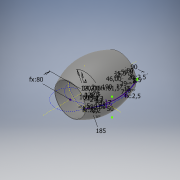
# Autodesk Inventor part: Form
Saved by Autodesk Inventor 2018.3 (Build 223284000, 284)
## iProperties
Created: 2018-07-22
Part Number: Form
Material: Generisch
Document SubType Name: Modeling
Designer: JochenAlt
Density: 1 g/cm^3
Appearance: Textur - grau
Author: JochenAlt
Autodesk Inventor part; units mm, degrees
ref_plane "YZ Plane" through (0, 0, 0) normal (1, 0, 0) x (0, 1, 0)
ref_plane "XY Plane" through (0, 0, 0) normal (0, 0, 1) x (1, 0, 0)
sketch "Skizze3" plane through (0, 0, 0) normal (0, 0, 1) x (1, 0, 0)
  line L0 (0, 284.3849) -> (0, -234.0642) construction
  line L1 (-127.25, 0) -> (203.5, 0) construction
  line L2 (92.5, 190) -> (90, 190)
  circle A0 centre (0, 0) radius 80 construction
  circle A1 centre (0, -80) radius 80 construction
  line L3 (83, -80) -> (85.5, -80)
  line L4 (83, -80) -> (131.774, 9.2102) construction
  line L5 (131.774, 94.6678) -> (90, 190) construction
  spline S0 degree 3 poles (83, -80) (131.774, 9.2102) (131.774, 94.6678) (90, 190) knots 1 1 1 1 2 2 2 2
  line L6 (92.5, 190) -> (133.774, 95.8088) construction
  line L7 (133.774, 8.2956) -> (85.5, -80) construction
  spline S1 degree 3 poles (92.5, 190) (133.774, 95.8088) (133.774, 8.2956) (85.5, -80) knots 1 1 1 1 2 2 2 2
  line L8 (153.75, 101.6438) -> (156.25, 101.6438) construction
  line L9 (153.75, 101.6438) -> (156.25, 101.6438) construction
  line L10 (133.774, 95.8088) -> (133.774, 8.2956) construction
  line L11 (131.774, 9.2102) -> (131.774, 94.6678) construction
  line L12 (57.5472, 55.5727) -> (101.7866, 98.2942) construction
  line L13 (57.5472, -24.4273) -> (101.7866, 18.2942) construction
  circle A2 centre (101.7866, 18.2942) radius 8.5 construction
  circle A3 centre (101.7866, 98.2942) radius 8.5 construction
  line L14 (83, -80) -> (80, -80) construction
  line L15 (110.1767, 16.9319) -> (117.0862, 15.81) construction
  line L16 (110.1836, 99.6135) -> (117.0987, 100.7) construction
  line L17 (109.0162, 129.7466) -> (110.9529, 130.2457) construction
  arc A4 (104.9108, 115.2128) -> (105.281, 136.4227) centre (94.4909, 126.0029) ccw construction
  line L18 (105.281, 136.4227) -> (51.2009, 192.4243) construction
  line L19 (104.9108, 115.2128) -> (67.4188, 79.0073) construction
  line L20 (92.5, 190) -> (88.2437, 199.7132) construction
  line L21 (88.2437, 199.7132) -> (82.5, 210) construction
  spline S2 degree 2 poles (92.5, 190) (88.2437, 199.7132) (82.5, 210) knots 1 1 1 2 2 2
  line L22 (90, 190) -> (85.7437, 199.7132) construction
  line L23 (85.7437, 199.7132) -> (80, 210) construction
  spline S3 degree 2 poles (90, 190) (85.7437, 199.7132) (80, 210) knots 1 1 1 2 2 2
  line L24 (82.5, 210) -> (80, 210)
  line L25 (90, 190) -> (90, 185)
  line L26 (90, 185) -> (88, 185)
  line L27 (88, 185) -> (88, 183)
  line L28 (88, 183) -> (92.9995, 183)
  line L29 (90, 190) -> (59.8, 190) construction
  line L30 (59.8, 190) -> (59.8, 185)
  line L31 (59.8, 185) -> (22, 172.5)
  arc A5 (49.9582, 183.7454) -> (59.8, 190) centre (42.4636, 206.409) ccw
  line L32 (49.9582, 183.7454) -> (22, 174.5)
  line L33 (22, 174.5) -> (22, 172.5)
  line L34 (59.8, 185) -> (88, 185) construction
  line L35 (22, 174.5) -> (9.0124, 174.5)
  line L36 (9.0124, 174.5) -> (9.0124, 172.5)
  line L37 (9.0124, 172.5) -> (22, 172.5)
  point P0 (90, 149.8145)
  point P1 (22, 173.5)
  dimension "d13" = 160
  dimension "d108" = 17
  dimension "d7" = 190
  dimension "d11" = 2.5
  dimension "d14" = 80
  dimension "d15" = 90
  dimension "d18" = 2.5
  dimension "d19" = 2.5
  dimension "d105" = 2
  dimension "d106" = 61.5
  dimension "d107" = 46
  dimension "d110" = 3
  dimension "d111" = 7
  dimension "d112" = 7
  dimension "d119" = 10
  dimension "d120" = 15
  dimension "d121" = 29
  dimension "d122" = 2
  dimension "d127" = 2.5
  dimension "d128" = 80
  dimension "d129" = 20
  dimension "d137" = 5
  dimension "d149" = 2
  dimension "d181" = 2
  dimension "d183" = 59.8
  dimension "d184" = 22
  dimension "d185" = 15.5
  constraints: 52 end point, 10 horizontal, 9 point on circle, 8 parallel, 5 point on line, 4 perpendicular, 3 centre point, 3 equal length, 3 tangent, 3 vertical, 2 coincident, 2 line through centre, 1 collinear, 1 midpoint, 31 other
  measures "d7" distance between parallel lines of L1 L2
  measures "d11" distance of L2.start L2.end
  measures "d14" distance of A1.centre point (0, 0)
  measures "d15" distance from line of L0 L2.end
  measures "d18" distance of L3.end L3.start
  measures "d19" distance of L8.start L8.end
  measures "d105" distance between parallel lines of L10 L11
  measures "d106" distance of L12.start L12.end
  measures "d107" angle of L0 L12
  measures "d110" distance of L3.start L14.end
  measures "d111" distance of L15.start L15.end
  measures "d112" distance of L16.start L16.end
  measures "d119" distance from line of L19.start L12
  measures "d120" radius of A4
  measures "d121" distance from line of L18 point (101.787, 98.294)
  measures "d122" distance of L17.start L17.end
  measures "d127" distance of L21.end L23.end
  measures "d128" distance from line of L0 L23.end
  measures "d129" distance between parallel lines of L2 L24
  measures "d137" distance of L2.end L25.end
  measures "d149" distance of L26.end L27.end
  measures "d181" distance of L31.end L32.end
  measures "d183" distance between parallel lines of L30 L0
  measures "d184" distance between parallel lines of L0 L33
  measures "d185" distance between parallel lines of L35 L29
revolve "Umdrehung1" add sketch "Skizze3" angle 360 about axis through (0, 0, 0) along (0, -1, 0) contours S1 L3 S0 L2 | S0 L28 L27 L26 L25
sketch "Skizze6" plane through (0, 0, 0) normal (1, 0, 0) x (0, 1, 0)
  line L0 (-38, 0) -> (228, 0) construction
  line L1 (0, 126) -> (0, -126) construction
  line L2 (158.5, 25) -> (158.5, -25)
  line L3 (168.5, 25) -> (158.5, 25)
  line L4 (158.5, -25) -> (168.5, -25)
  line L5 (168.5, -25) -> (168.5, 25)
  line L6 (190, 90) -> (190, -90) projected
  point P0 (0, 0)
  point P1 (190, 0)
  dimension "d35" = 50
  dimension "d49" = 21.5
  dimension "d51" = 10
  constraints: 8 end point, 2 vertical, 1 horizontal, 1 parallel, 1 other
  measures "d35" distance of L2.start L2.end
  measures "d49" distance between parallel lines of L6 L5
  measures "d51" distance of L2.end L4.end
extrude "Extrusion4" add sketch "Skizze6" along normal up to next separate body
sketch "Skizze7" plane through (0, 0, 0) normal (0, 1, 0) x (-1, 0, 0)
  arc A0 (-91.5321, 13.3464) -> (-91.5321, -13.3464) centre (0, 0) ccw
  circle A1 centre (-70, 0) radius 7.6
  line L0 (-68.5427, -9.9943) -> (-91.5321, -13.3464)
  line L1 (-68.5427, 9.9943) -> (-91.5321, 13.3464)
  line L2 (-92.5, 0) -> (-122.6318, 0) construction
  arc A2 (-68.5427, -9.9943) -> (-68.5427, 9.9943) centre (-70, 0) ccw
  circle A3 centre (-70, 0) radius 6.6
  line L3 (-91.5321, -13.3464) -> (-120, -17.4974)
  line L4 (-91.5321, 13.3464) -> (-120, 17.4974)
  line L5 (-120, -17.4974) -> (-120, 17.4974)
  arc A4 (-44.9, 77.7691) -> (-44.9, -77.7691) centre (0, 0) ccw
  line L6 (-44.9, -77.7691) -> (-37.4, -64.7787)
  line L7 (-44.9, 77.7691) -> (-38.4, 66.5108)
  line L8 (-190.011, 0) -> (136.6685, 0) construction
  circle A5 centre (0, 0) radius 85 construction
  circle A6 centre (0, 0) radius 90 construction
  circle A7 centre (-82, 0) radius 1.15
  circle A8 centre (-82, 0) radius 2.15 construction
  line L9 (-84.15, 1.2413) -> (-82, 2.4826)
  line L10 (-82, 2.4826) -> (-79.85, 1.2413)
  line L11 (-79.85, 1.2413) -> (-79.85, -1.2413)
  line L12 (-79.85, -1.2413) -> (-82, -2.4826)
  line L13 (-82, -2.4826) -> (-84.15, -1.2413)
  line L14 (-84.15, -1.2413) -> (-84.15, 1.2413)
  line L15 (0, -126) -> (0, 126) construction
  line L16 (-37.4, -64.7787) -> (0, 0)
  line L17 (-38.4, 66.5108) -> (0, 0)
  arc A9 (-43.9, 76.037) -> (-43.9, -76.037) centre (0, 0) ccw
  circle A10 centre (-35.764, 0) radius 12.7
  circle A11 centre (-35.764, 0) radius 8.5 construction
  circle A12 centre (-35.764, -8.5) radius 1.65
  circle A13 centre (-35.764, 8.5) radius 1.65
  circle A14 centre (-35.764, 0) radius 14.7
  circle A15 centre (-35.764, 0) radius 4
  line L18 (-35.764, 8.5) -> (-35.764, -8.5) construction
  line L19 (-37.2327, -16.8177) -> (-37.0429, -14.6443) construction
  line L20 (0, -25) -> (0, 25) projected
  line L21 (-68.4599, -30.1378) -> (-70.2903, -30.9436)
  line L22 (-68.4599, 30.1378) -> (-70.2903, 30.9436)
  arc A16 (-55.468, 53.1182) -> (-70.2903, 30.9436) centre (0, 0) ccw
  arc A17 (-70.2903, -30.9436) -> (-55.468, -53.1182) centre (0, 0) ccw
  line L23 (-54.0235, 51.7349) -> (-55.468, 53.1182)
  line L24 (-54.0235, -51.7349) -> (-55.468, -53.1182)
  arc A18 (-54.0235, 51.7349) -> (-68.4599, 30.1378) centre (0, 0) ccw
  arc A19 (-68.4599, -30.1378) -> (-54.0235, -51.7349) centre (0, 0) ccw
  arc A20 (-68.3984, -10.9839) -> (-68.3984, 10.9839) centre (-70, 0) ccw
  line L25 (-68.3984, -10.9839) -> (-73.8664, -11.7811)
  line L26 (-68.3984, 10.9839) -> (-73.8664, 11.7811)
  line L27 (-38.4, 66.5108) -> (-37.4, 64.7787)
  line L28 (-37.4, -64.7787) -> (-37.4, -64.7787)
  line L29 (-70.2903, 30.9436) -> (-68.4599, 30.1378)
  arc A21 (-41.6465, 62.1338) -> (-54.0235, 51.7349) centre (0, 0) ccw
  arc A22 (-54.0235, -51.7349) -> (-41.6465, -62.1338) centre (0, 0) ccw
  arc A23 (-68.4599, 30.1378) -> (-73.8664, 11.7811) centre (0, 0) ccw
  arc A24 (-73.8664, -11.7811) -> (-68.4599, -30.1378) centre (0, 0) ccw
  arc A25 (-50.4421, 0.8014) -> (-68.4599, 30.1378) centre (-80.6485, 2.4506) ccw
  arc A26 (-68.4599, -30.1378) -> (-50.4421, -0.8014) centre (-80.6485, -2.4506) ccw
  line L30 (-41.6465, -62.1338) -> (-11.0336, -9.1107)
  line L31 (-11.0336, 9.1107) -> (-41.6465, 62.1338)
  arc A27 (-54.0235, -51.7349) -> (-22.2402, -5.7617) centre (-150.294, 48.7943) ccw
  arc A28 (-22.2402, 5.7617) -> (-54.0235, 51.7349) centre (-150.294, -48.7943) ccw
  arc A29 (-11.0336, 9.1107) -> (-11.0336, -9.1107) centre (0, 0) ccw
  point P0 (-90, 0)
  point P1 (-85.5, 0)
  point P2 (-84.15, 0)
  point P3 (-21.064, 0)
  point P4 (-5.7735, 0)
  dimension "d132" = 4.3
  dimension "d32" = 185
  dimension "d40" = 15.2
  dimension "d53" = 1
  dimension "d56" = 50
  dimension "d101" = 170
  dimension "d116" = 0.2
  dimension "d130" = 2.3
  dimension "d140" = 2.5
  dimension "d141" = 120
  dimension "d142" = 70
  dimension "d148" = 12
  dimension "d150" = 25.4
  dimension "d151" = 17
  dimension "d152" = 3.3
  dimension "d153" = 2
  dimension "d154" = 8
  dimension "d159" = 34.236
  dimension "d187" = 20
  dimension "d188" = 1
  dimension "d189" = 2
  dimension "d192" = 15
  dimension "d194" = 2
  dimension "d195" = 5
  constraints: 56 end point, 47 point on circle, 28 centre point, 17 coincident, 16 tangent, 11 point on line, 5 equal length, 4 collinear, 3 midpoint, 3 parallel, 2 concentric, 2 horizontal alignment, 2 vertical, 1 equal radius, 1 line through centre, 22 other
  measures "d32" diameter of A0
  measures "d40" diameter of A1
  measures "d53" radial gap between concentric circles of A3 A1
  measures "d56" distance from line of L5 A1.centre
  measures "d101" diameter of A5
  measures "d130" diameter of A7
  measures "d140" radial gap between concentric circles of A2 A1
  measures "d141" angle of L17 L16
  measures "d142" distance of A2.centre L16.end
  measures "d148" distance of A7.centre A1.centre
  measures "d150" diameter of A10
  measures "d151" diameter of A11
  measures "d152" diameter of A12
  measures "d153" radial gap between concentric circles of A14 A10
  measures "d154" diameter of A15
  measures "d159" distance of A10.centre A1.centre
  measures "d187" angle of L21 L24
  measures "d188" radial gap between concentric circles of A20 A2
  measures "d189" radial gap between concentric circles of A18 A16
  measures "d192" radial gap between concentric circles of A24 A4
  measures "d194" radial gap between concentric circles of A4 A9
  measures "d195" distance between parallel lines of L30 L16
extrude "Extrusion5" cut sketch "Skizze7" along normal through all both and the other way through all contours L1 A4 L0 A0 | A0 L3 L5 L4 | L1 A9 L0 A4 | L1 A2 L0 A9 | L9 L10 L11 L12 L13 L14 keep common part bodies 2
extrude "Extrusion8" add sketch "Skizze7" along normal blind 7 from surface at 158.5 contours A1 bodies 2
extrude "Extrusion9" add sketch "Skizze7" along normal blind 1 from surface at 158.5 contours A1 bodies 2
extrude "Extrusion16" cut sketch "Skizze7" along normal blind 5 from surface at 158.5 contours A7 | L9 L10 L11 L12 L13 L14 bodies 1 2
pattern_circular "Runde Anordnung2" count 3 over 360 about axis through (0, -10, 0) along (0, 1, 0) bodies 2
combine bodies "Kombinieren2" operation type add bodies to combine 2 1
extrude "Extrusion10" add sketch "Skizze7" against normal blind 1 from surface at 190 separate body contours A4 L7 A9 L1 | L1 A9 L0 A4 | L0 A9 L6 A4 | A9 L7 L17 L16 L6 L0 A2 L1 | L1 A2 L0 A9 | A1 | L9 L10 L11 L12 L13 L14 | A18 L22 A16 L23 | L24 A17 L21 A19
extrude "Extrusion11" add sketch "Skizze7" against normal blind 4 from surface at 189 contours A4 L7 A9 L1 | L1 A9 L0 A4 | L0 A9 L6 A4 | A9 L7 L17 L16 L6 L0 A2 L1 | L1 A2 L0 A9 | L9 L10 L11 L12 L13 L14 | A18 L22 A16 L23 | L24 A17 L21 A19 bodies 3
extrude "Extrusion17" cut sketch "Skizze7" against normal blind 2 from surface at 190 contours A4 L7 A9 L1 | L1 A9 L0 A4 | L0 A9 L6 A4 bodies 3
pattern_circular "Runde Anordnung3" count 3 over 360 about axis through (0, -10, 0) along (0, 1, 0) of "Extrusion10", "Extrusion11", "Extrusion17" bodies 3
ref_plane "MotorGear" through (70, 174.5, 0) normal (0, 1, 0) x (1, 0, 0)
extrude "Extrusion18" add sketch "Skizze7" against normal blind 2 from surface at 174.5 contours A10 | A14 | A14 A25 A18 A28 | A27 A19 A26 A14 | A18 L22 A16 L23 | L24 A17 L21 A19 bodies 3
extrude "Extrusion19" add sketch "Skizze7" against normal blind 5 from surface at 174.5 contours A14 bodies 3
extrude "Extrusion21" add sketch "Skizze7" along normal up to surface (10.5 mm away) from surface at 174.5 contours A18 L22 A16 L23 | L24 A17 L21 A19 bodies 3
fillet "Rundung3" radius 10 2 edges at (62.1864, 174.5, 41.5679) (62.1864, 174.5, -41.5679)
fillet "Rundung4" radius 12 2 edges at (63.8492, 172.5, -42.6793) (63.8492, 172.5, 42.6793)
sketch "Schnnitt" plane through (0, 50, 0) normal (0, 1, 0) x (-1, 0, 0)
  line L0 (0, 0) -> (161.4612, 0)
  line L1 (0, 0) -> (-80.7306, 139.8295)
  line L2 (0, 0) -> (-80.7306, -139.8295)
  circle A0 centre (0, 0) radius 161.4612
  line L3 (226.0456, 0) -> (-226.0456, 0) construction
  line L4 (0, -226.0456) -> (0, 226.0456) construction
  dimension "d123" = 120
  constraints: 6 end point, 3 point on circle, 1 centre point, 1 coincident, 1 horizontal, 1 other
  measures "d123" angle of L2 L1
equation "\"d14\" = 0.5 * d13"
equation "\"d18\" = d17"
equation "\"d16\" = d11"
equation "\"d17\" = d16"
